Autodesk Fusion 360 part; units mm, degrees
(part 2 of 2)
  spline S106 degree 3 poles (-4.8701, -8.0877) (-4.8678, -8.1149) (-4.8633, -8.1695) (-4.8329, -8.2151) (-4.8175, -8.2381) knots 0 0 0 0 0.008046 0.016168 0.016168 0.016168 0.016168
  spline S107 degree 3 poles (-4.8175, -8.2381) (-4.7961, -8.2607) (-4.7493, -8.3102) (-4.6868, -8.3377) (-4.6528, -8.3527) knots 0 0 0 0 0.009247 0.020247 0.020247 0.020247 0.020247
  spline S108 degree 3 poles (-4.6528, -8.3527) (-4.6105, -8.366) (-4.4848, -8.4056) (-4.3576, -8.4398) (-4.2732, -8.4625) knots 0 0 0 0 0.01331 0.039521 0.039521 0.039521 0.039521
  spline S109 degree 3 poles (-4.2732, -8.4625) (-4.1434, -8.497) (-3.9283, -8.5541) (-3.7197, -8.6312) (-3.6369, -8.6618) knots 0 0 0 0 0.040259 0.066707 0.066707 0.066707 0.066707
  spline S110 degree 3 poles (-3.6369, -8.6618) (-3.5805, -8.6901) (-3.4701, -8.7452) (-3.3921, -8.8408) (-3.354, -8.8874) knots 0 0 0 0 0.018692 0.036554 0.036554 0.036554 0.036554
  spline S111 degree 3 poles (-3.354, -8.8874) (-3.3241, -8.9415) (-3.2609, -9.0557) (-3.2547, -9.1864) (-3.2514, -9.2551) knots 0 0 0 0 0.018292 0.038629 0.038629 0.038629 0.038629
  spline S112 degree 3 poles (-3.2514, -9.2551) (-3.2569, -9.3262) (-3.2681, -9.4704) (-3.3402, -9.596) (-3.3767, -9.6598) knots 0 0 0 0 0.021094 0.042838 0.042838 0.042838 0.042838
  spline S113 degree 3 poles (-3.3767, -9.6598) (-3.4244, -9.72) (-3.523, -9.8446) (-3.665, -9.9164) (-3.7384, -9.9534) knots 0 0 0 0 0.022753 0.047089 0.047089 0.047089 0.047089
  spline S114 degree 3 poles (-3.7384, -9.9534) (-3.8215, -9.9837) (-3.9942, -10.0466) (-4.1779, -10.0537) (-4.2732, -10.0573) knots 0 0 0 0 0.026364 0.054775 0.054775 0.054775 0.054775
  line L53 (-1.875, -15.7441) -> (0, -13.8691)
  line L54 (-25.5, -13.8691) -> (-23.625, -15.7441)
  line L55 (-23.625, -15.7441) -> (-12.75, -18.6581)
  line L56 (-12.75, -18.6581) -> (-1.875, -15.7441)
  circle A1 centre (-12.75, -15.2374) radius 1.4264
  dimension "d95" = 5.4528
  constraint coincident A0.centre A1.centre
  measures "d95" diameter of A0
extrude "Countersink Cutout" cut sketch "Countersink" against normal blind 3 contours A0 | A1
sketch "Sketch6" plane through (-70, 0, 0) normal (-1, 0, 0) x (0, -1, 0)
  line L0 (0, -13.8691) -> (1.875, -15.7441)
  line L1 (1.875, -15.7441) -> (12.75, -18.6581)
  line L2 (12.75, -18.6581) -> (23.625, -15.7441)
  line L3 (23.625, -15.7441) -> (25.5, -13.8691)
  line L4 (25.5, -13.8691) -> (25.5, 0)
  line L5 (25.5, 0) -> (0, 0)
  line L6 (0, 0) -> (0, -13.8691)
  line L7 (2.1, 0) -> (23.4, 0)
  line L8 (23.4, 0) -> (23.4, -13)
  line L9 (23.4, -13) -> (2.1, -13)
  line L10 (2.1, -13) -> (2.1, 0)
  line L11 (3.75, 0) -> (21.75, 0)
  line L12 (21.75, 0) -> (21.75, -13)
  line L13 (21.75, -13) -> (3.75, -13)
  line L14 (3.75, -13) -> (3.75, 0)
  line L15 (2.1, 0) -> (3.75, -13)
  line L16 (23.4, 0) -> (21.75, -13)
  circle A0 centre (12.75, -15.2374) radius 1.4264
  dimension "d29" = 21.3
  dimension "d31" = 2.1
  dimension "d36" = 18
  dimension "d37" = 1.65
  dimension "d40" = 13
  constraint horizontal L7
  constraint vertical L8
  constraint horizontal L9
  constraint vertical L10
  constraint collinear L5 L7
  constraint horizontal L11
  constraint vertical L12
  constraint horizontal L13
  constraint vertical L14
  constraint coincident L9 L12.end
  constraint coincident L7 L11.start
  measures "d29" distance of L7.start L7.end
  measures "d31" distance of L6 L10
  measures "d36" distance of L12 L14
  measures "d37" distance of L10 L14
  measures "d40" distance of L7 L9
extrude "Extrude5" cut sketch "Sketch6" against normal blind 1 from surface at -1 contours L9 L10 L15 | L5 L7 L14 L15 | L5 L7 L9 L11 L12 L13 L14 | L5 L7 L12 L16 | L8 L9 L16
extrude "Extrude6" cut sketch "Sketch6" against normal blind 1 contours L5 L7 L14 L15 | L5 L7 L9 L11 L12 L13 L14 | L5 L7 L12 L16
sketch "Sketch7" plane through (0, 0, 0) normal (0, 0, 1) x (-1, 0, 0)
  line L0 (70, 23.4) -> (70, 25.5)
  line L1 (70, 25.5) -> (62, 25.5)
  line L2 (62, 25.5) -> (62, 0)
  line L3 (62, 0) -> (70, 0)
  line L4 (69, 2.1) -> (68, 2.1)
  line L5 (68, 2.1) -> (68, 23.4)
  line L6 (68, 23.4) -> (69, 23.4)
  line L7 (63.85, 20) -> (63.85, 5.5)
  arc A0 (63.85, 5.5) -> (66.85, 5.5) centre (65.35, 5.5) ccw
  line L8 (66.85, 5.5) -> (66.85, 20)
  arc A1 (66.85, 20) -> (63.85, 20) centre (65.35, 20) ccw
  line L9 (65.35, 20) -> (65.35, 5.5) construction
  line L10 (70, 2.1) -> (69, 2.1)
  line L11 (69, 23.4) -> (70, 23.4)
  line L12 (70, 0) -> (70, 2.1)
  point P0 (65.35, 12.75)
  dimension "d41" = 12.75
  dimension "d42" = 3.35
  dimension "d43" = 1.5
  dimension "d44" = 14.5
  constraint tangent L7 A0
  constraint tangent A0 L8
  constraint parallel L7 L8
  constraint tangent L8 A1
  constraint tangent L7 A1
  constraint parallel L2 L9
  constraint midpoint L9 P0
  measures "d41" distance of L1 P0
  measures "d42" distance of L2 P0
  measures "d43" radius of A0
  measures "d44" distance of L7.start L7.end
extrude "Extrude7" add sketch "Sketch7" along normal blind 1 contours L7 A0 L8 A1
fillet "Fillet2" radius 1 tangency weight 0.81441 4 edges at (-66.85, -12.75, 1) (-65.35, -21.5, 1) (-63.85, -12.75, 1) (-65.35, -4, 1)
sketch "Sketch8" plane through (-68, 0, 0) normal (-1, 0, 0) x (0, -1, 0)
  line L0 (2.1, -13) -> (23.4, -13)
  line L1 (23.4, -13) -> (23.4, 0)
  line L2 (23.4, 0) -> (2.1, 0)
  line L3 (2.1, 0) -> (2.1, -13)
  line L4 (10.17, -13) -> (10.17, -12.4)
  line L5 (10.67, -11.9) -> (11.77, -11.9)
  line L6 (12.27, -11.4) -> (12.27, -7.02)
  line L7 (12.77, -6.52) -> (12.97, -6.52)
  line L8 (13.47, -7.02) -> (13.47, -11.4)
  line L9 (13.97, -11.9) -> (15.07, -11.9)
  line L10 (15.57, -12.4) -> (15.57, -13)
  arc A0 (12.77, -6.52) -> (12.27, -7.02) centre (12.77, -7.02) ccw
  arc A1 (13.47, -7.02) -> (12.97, -6.52) centre (12.97, -7.02) ccw
  arc A2 (13.47, -11.4) -> (13.97, -11.9) centre (13.97, -11.4) ccw
  arc A3 (15.57, -12.4) -> (15.07, -11.9) centre (15.07, -12.4) ccw
  arc A4 (11.77, -11.9) -> (12.27, -11.4) centre (11.77, -11.4) ccw
  arc A5 (10.67, -11.9) -> (10.17, -12.4) centre (10.67, -12.4) ccw
  point P0 (12.75, -13)
  dimension "d49" = 0.5
  dimension "d50" = 4.38
  dimension "d51" = 0.2
  dimension "d52" = 1.1
  dimension "d53" = 0.6
  dimension "d54" = 0.6
  dimension "d55" = 2.58
  dimension "d56" = 1.1
  constraint coincident L0 L4.start
  constraint perpendicular L0 L4
  constraint perpendicular L4 L5
  constraint perpendicular L5 L6
  constraint perpendicular L6 L7
  constraint perpendicular L5 L8
  constraint perpendicular L6 L9
  constraint coincident L0 L10.end
  constraint perpendicular L0 L10
  constraint tangent L7 A0
  constraint tangent L6 A0
  constraint tangent L7 A1
  constraint tangent L8 A1
  constraint equal A0 A1
  constraint tangent L8 A2
  constraint tangent L9 A2
  constraint equal A0 A2
  constraint tangent L9 A3
  constraint tangent L10 A3
  constraint equal A0 A3
  constraint tangent L5 A4
  constraint tangent L6 A4
  constraint equal A0 A4
  constraint tangent L5 A5
  constraint tangent L4 A5
  constraint equal A0 A5
  constraint midpoint L0 P0
  measures "d49" radius of A0
  measures "d50" distance of L6.end L6.start
  measures "d51" distance of L7.start L7.end
  measures "d52" distance of L9.start L9.end
  measures "d53" distance of L10.end L10.start
  measures "d54" distance of L4.start L4.end
  measures "d55" distance of L4.start P0
  measures "d56" distance of L5.end L5.start
extrude "Extrude8" add sketch "Sketch8" along normal blind 2 contours L0 L4 L5 L6 L7 L8 L9 L10 A0 A1 A2 A3 A4 A5
sketch "Sketch9" plane through (-68, 0, 0) normal (-1, 0, 0) x (0, -1, 0)
  line L0 (10.17, -13) -> (10.17, -12.4)
  arc A0 (10.67, -11.9) -> (10.17, -12.4) centre (10.67, -12.4) ccw
  line L1 (10.67, -11.9) -> (11.77, -11.9)
  arc A1 (11.77, -11.9) -> (12.27, -11.4) centre (11.77, -11.4) ccw
  line L2 (12.27, -11.4) -> (12.27, -7.02)
  arc A2 (12.77, -6.52) -> (12.27, -7.02) centre (12.77, -7.02) ccw
  line L3 (12.77, -6.52) -> (12.97, -6.52)
  arc A3 (13.47, -7.02) -> (12.97, -6.52) centre (12.97, -7.02) ccw
  line L4 (13.47, -7.02) -> (13.47, -11.4)
  arc A4 (13.47, -11.4) -> (13.97, -11.9) centre (13.97, -11.4) ccw
  line L5 (13.97, -11.9) -> (15.07, -11.9)
  arc A5 (15.57, -12.4) -> (15.07, -11.9) centre (15.07, -12.4) ccw
  line L6 (15.57, -12.4) -> (15.57, -13)
  line L7 (15.57, -13) -> (23.4, -13)
  line L8 (23.4, -13) -> (23.4, 0)
  line L9 (23.4, 0) -> (2.1, 0)
  line L10 (2.1, 0) -> (2.1, -13)
  line L11 (2.1, -13) -> (10.17, -13)
  line L12 (6.07, -8.4) -> (9.27, -8.4)
  line L13 (9.27, -8.4) -> (9.27, -10.15)
  line L14 (9.27, -10.15) -> (6.07, -10.15)
  line L15 (6.07, -10.15) -> (6.07, -8.4)
  line L16 (16.47, -8.4) -> (19.67, -8.4)
  line L17 (19.67, -8.4) -> (19.67, -10.15)
  line L18 (19.67, -10.15) -> (16.47, -10.15)
  line L19 (16.47, -10.15) -> (16.47, -8.4)
  dimension "d59" = 3.2
  dimension "d60" = 1.75
  dimension "d61" = 8.4
  dimension "d62" = 3
  dimension "d63" = 3.2
  dimension "d64" = 1.75
  dimension "d65" = 8.4
  dimension "d66" = 3
  constraint horizontal L12
  constraint vertical L13
  constraint horizontal L14
  constraint vertical L15
  constraint horizontal L16
  constraint vertical L17
  constraint horizontal L18
  constraint vertical L19
  measures "d59" distance of L12.start L12.end
  measures "d60" distance of L12.start L14.end
  measures "d61" distance of L9 L12
  measures "d62" distance of L2 L13
  measures "d63" distance of L16.start L16.end
  measures "d64" distance of L16.start L18.end
  measures "d65" distance of L9 L16
  measures "d66" distance of L4 L19
extrude "Extrude9" cut sketch "Sketch9" against normal blind 1 contours L12 L13 L14 L15 | L16 L17 L18 L19
fillet "Fillet3" radius 1 2 edges at (-68, -7.67, -8.4) (-68, -18.07, -8.4)
equation "d63 = d59"
equation "d64 = d60"
equation "d65 = d61"
equation "d66 = d62"
equation "d76 = d75"
equation "d78 = d77"
equation "d83 = d84"
named bodies: "Battery_Cap"
